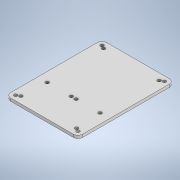
# Autodesk Inventor part: EboxMounting_Plate
Saved by Autodesk Inventor 2021 (Build 250183000, 183)
## iProperties
Created: 2021-10-09
Part Number: EboxMounting_Plate
Material: Generic
Document SubType Name: Modeling
Designer: Jorian Brusind
Density: 1 g/cm^3
Appearance: Default
Author: Jorian Brusind
Autodesk Inventor part; units mm, degrees
ref_plane "YZ Plane" through (0, 0, 0) normal (1, 0, 0) x (0, 1, 0)
ref_plane "XZ Plane" through (0, 0, 0) normal (0, 1, 0) x (-1, 0, 0)
ref_plane "XY Plane" through (0, 0, 0) normal (0, 0, 1) x (1, 0, 0)
sketch "Sketch2" plane through (0, 0, 0) normal (0, 1, 0) x (-1, 0, 0)
  line L0 (0, 0) -> (75, 0)
  line L1 (75, 0) -> (75, -100)
  line L2 (75, -100) -> (0, -100)
  line L3 (0, -100) -> (0, 0)
  circle A0 centre (70, -5) radius 1.75
  circle A1 centre (70, -95) radius 1.75
  circle A2 centre (5, -5) radius 1.75
  circle A3 centre (5, -95) radius 1.75
  circle A4 centre (65, -33) radius 1.75
  circle A5 centre (40, -33) radius 1.75
  circle A6 centre (66.5, -7) radius 1.75
  circle A7 centre (66.5, -93) radius 1.75
  circle A8 centre (8.5, -7) radius 1.75
  circle A9 centre (8.5, -93) radius 1.75
  line L4 (37.5, 0) -> (37.5, -100)
  circle A10 centre (10, -33) radius 1.75
  circle A11 centre (35, -33) radius 1.75
  dimension "d13" = 75
  dimension "d14" = 100
  dimension "d15" = 3.5
  dimension "d16" = 5
  dimension "d17" = 5
  dimension "d20" = 90
  dimension "d23" = 65
  dimension "d26" = 3.5
  dimension "d27" = 10
  dimension "d28" = 33
  dimension "d29" = 3.5
  dimension "d30" = 25
  dimension "d31" = 33
  dimension "d32" = 3.5
  dimension "d35" = 86
  dimension "d38" = 58
  dimension "d41" = 8.5
  dimension "d42" = 7
  constraints: 12 centre point, 10 end point, 3 horizontal, 2 midpoint, 2 parallel, 2 symmetric about line, 2 vertical, 1 perpendicular, 14 other
  measures "d13" distance of L1.end L2.end
  measures "d14" distance of L0.end L1.end
  measures "d15" diameter of A0
  measures "d16" distance from line of L1 A0.centre
  measures "d17" distance from line of L0 A0.centre
  measures "d20" distance of A0.centre A1.centre
  measures "d23" distance of A0.centre A2.centre
  measures "d26" diameter of A4
  measures "d27" distance from line of L1 A4.centre
  measures "d28" distance from line of L0 A4.centre
  measures "d29" diameter of A5
  measures "d30" distance of A5.centre A4.centre
  measures "d31" distance from line of L0 A5.centre
  measures "d32" diameter of A6
  measures "d35" distance of A6.centre A7.centre
  measures "d38" distance of A6.centre A8.centre
  measures "d41" distance from line of L1 A6.centre
  measures "d42" distance from line of L0 A6.centre
extrude "Extrusion2" add sketch "Sketch2" along normal blind 3
fillet "Fillet2" radius 5 4 edges at (0, 1.5, -100) (-75, 1.5, -100) (0, 1.5, 0) (-75, 1.5, 0)
body "Solid2"
